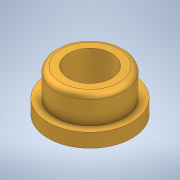
# Autodesk Inventor part: bøsning_beslag_3D
Saved by Autodesk Inventor 2022 (Build 260153000, 153)
## iProperties
Created: 2022-04-10
Part Number: bøsning_beslag_3D
Material: Brass, Soft Yellow
Document SubType Name: Modeling
Designer: Patrick
Density: 8.47 g/cm^3
Appearance: Brass - Satin
Mass: 2.90673 g
Surface Area: 4.71068 cm^2
Volume: 0.34318 cm^3
Author: Patrick
Autodesk Inventor part; units mm, degrees
ref_plane "YZ Plane" through (0, 0, 0) normal (1, 0, 0) x (0, 1, 0)
ref_plane "XZ Plane" through (0, 0, 0) normal (0, 1, 0) x (-1, 0, 0)
ref_plane "XY Plane" through (0, 0, 0) normal (0, 0, 1) x (1, 0, 0)
sketch "Sketch1" plane through (0, 0, 0) normal (0, 1, 0) x (-1, 0, 0)
  circle A0 centre (0, 0) radius 4.9
  circle A1 centre (0, 0) radius 3.1
  dimension "d0" = 9.8
  dimension "d1" = 6.2
  constraints: 2 centre point, 2 coincident
  measures "d0" diameter of A0
  measures "d1" diameter of A1
extrude "Extrusion1" add sketch "Sketch1" along normal blind 6
sketch "Sketch2" plane through (0, 0, 0) normal (0, -1, 0) x (1, 0, 0)
  circle A0 centre (0, 0) radius 6
  circle A1 centre (0, 0) radius 4.9 projected
  circle A2 centre (0, 0) radius 3.1 projected
  dimension "d4" = 12
  constraints: 1 centre point, 1 coincident
  measures "d4" diameter of A0
extrude "Extrusion2" add sketch "Sketch2" against normal blind 2 contours A0
fillet "Fillet1" radius 0.75 1 edges at (4.9, 6, 0)
body "Solid1"
